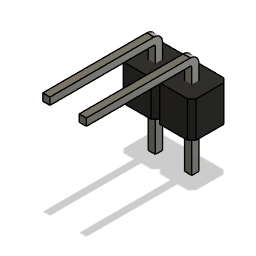
2.54mm 90 angle 2 pin header (Autodesk Fusion 360 design; units mm, degrees)
Autodesk Fusion 360 part; units mm, degrees
sketch "Sketch1" plane through (0, 0, 0) normal (0, 1, 0) x (1, 0, 0) in component "body"
  line L0 (0, 0) -> (-1.27, 0) construction
  line L1 (0, 0) -> (1.27, 0) construction
  line L2 (-0.0001, -1.27) -> (2.5401, -1.27)
  line L3 (2.5401, -1.27) -> (2.5401, 1.27)
  line L4 (2.5401, 1.27) -> (-0.0001, 1.27)
  line L5 (-0.0001, 1.27) -> (-0.0001, -1.27)
  line L6 (-0.0001, -1.27) -> (2.5401, 1.27) construction
  line L7 (2.5401, -1.27) -> (-0.0001, 1.27) construction
  line L8 (-0.0001, -1.27) -> (-2.5399, -1.27)
  line L9 (-2.5399, -1.27) -> (-2.5399, 1.27)
  line L10 (-2.5399, 1.27) -> (-0.0001, 1.27)
  line L11 (-0.0001, 1.27) -> (-0.0001, -1.27)
  line L12 (-0.0001, -1.27) -> (-2.5399, 1.27) construction
  line L13 (-2.5399, -1.27) -> (-0.0001, 1.27) construction
  point P0 (1.27, 0)
  point P1 (-1.27, 0)
  dimension "d1" = 1.27
  dimension "d2" = 1.27
  dimension "d3" = 2.54
  constraint coincident L0.start L1.start
  constraint horizontal L0
  constraint parallel L0 L1
  constraint horizontal L2
  constraint perpendicular L2 L3
  constraint parallel L2 L4
  constraint parallel L3 L5
  constraint coincident L6 P0
  constraint coincident L7 P0
  constraint coincident P0 L1.end
  constraint horizontal L8
  constraint perpendicular L8 L9
  constraint parallel L8 L10
  constraint parallel L9 L11
  constraint coincident L12 P1
  constraint coincident L13 P1
  constraint coincident P1 L0.end
  measures "d1" distance of L0.start L0.end
  measures "d2" distance of L0.start P0
  measures "d3" distance of L2.end L3.end
extrude "Extrude1" add sketch "Sketch1" along normal blind 2.5 contours L5 L8 L9 L10 L11 makes body 1 in component "body"
chamfer "Chamfer1" distance 0.3 angle 45 4 edges at (-0.0001, 1.25, 1.27) (-2.5399, 1.25, 1.27) (-0.0001, 1.25, -1.27) (-2.5399, 1.25, -1.27) on bodies 1 in component "body"
extrude "Extrude2" add sketch "Sketch1" along normal blind 2.5 contours L2 L3 L4 L5 L11 bodies 1 in component "body"
chamfer "Chamfer2" distance 0.3 angle 45 4 edges at (-0.0001, 1.25, 1.27) (2.5401, 1.25, 1.27) (2.5401, 1.25, -1.27) (-0.0001, 1.25, -1.27) on bodies 1 in component "body"
sketch "Sketch1 (2)" plane through (0, 2.5, 0) normal (0, 1, 0) x (-1, 0, 0) in component "pins"
  line L0 (-0.2999, -1.27) -> (0.0001, -0.97)
  line L1 (0.0001, -0.97) -> (0.3001, -1.27)
  line L2 (0.3001, -1.27) -> (2.2399, -1.27)
  line L3 (2.2399, -1.27) -> (2.5399, -0.97)
  line L4 (2.5399, -0.97) -> (2.5399, 0.97)
  line L5 (2.5399, 0.97) -> (2.2399, 1.27)
  line L6 (2.2399, 1.27) -> (0.3001, 1.27)
  line L7 (0.3001, 1.27) -> (0.0001, 0.97)
  line L8 (0.0001, 0.97) -> (-0.2999, 1.27)
  line L9 (-0.2999, 1.27) -> (-2.2401, 1.27)
  line L10 (-2.2401, 1.27) -> (-2.5401, 0.97)
  line L11 (-2.5401, 0.97) -> (-2.5401, -0.97)
  line L12 (-2.5401, -0.97) -> (-2.2401, -1.27)
  line L13 (-2.2401, -1.27) -> (-0.2999, -1.27)
  line L14 (-2.3901, -1.12) -> (-0.1499, 1.12) construction
  line L15 (0.1501, 1.12) -> (2.3899, -1.12) construction
  line L16 (-1.52, 0.25) -> (-1.02, 0.25)
  line L17 (-1.02, 0.25) -> (-1.02, -0.25)
  line L18 (-1.02, -0.25) -> (-1.52, -0.25)
  line L19 (-1.52, -0.25) -> (-1.52, 0.25)
  line L20 (-1.52, 0.25) -> (-1.02, -0.25) construction
  line L21 (-1.02, 0.25) -> (-1.52, -0.25) construction
  line L22 (1.02, 0.25) -> (1.52, 0.25)
  line L23 (1.52, 0.25) -> (1.52, -0.25)
  line L24 (1.52, -0.25) -> (1.02, -0.25)
  line L25 (1.02, -0.25) -> (1.02, 0.25)
  line L26 (1.02, 0.25) -> (1.52, -0.25) construction
  line L27 (1.52, 0.25) -> (1.02, -0.25) construction
  point P0 (-1.27, 0)
  point P1 (1.27, 0)
  dimension "d10" = 0.5
  dimension "d11" = 0.5
  constraint midpoint L12 L14.start
  constraint midpoint L8 L14.end
  constraint midpoint L7 L15.start
  constraint midpoint L3 L15.end
  constraint horizontal L16
  constraint perpendicular L16 L17
  constraint parallel L16 L18
  constraint parallel L17 L19
  constraint coincident L20 P0
  constraint coincident L21 P0
  constraint midpoint L14 P0
  constraint horizontal L22
  constraint perpendicular L22 L23
  constraint parallel L22 L24
  constraint parallel L23 L25
  constraint coincident L15 L22.start
  constraint coincident L26 P1
  constraint coincident L27 P1
  constraint midpoint L15 P1
  measures "d10" distance of L17.end L18.end
  measures "d11" distance of L16.end L17.end
extrude "Extrude1'" add sketch "Sketch1 (2)" against normal blind 5.5 separate body contours L16 L17 L18 L19 | L22 L23 L24 L25 makes body 2 at (1.02, 0.6667, 0.0833) makes body 3 at (-1.52, 0.6667, 0.0833) in component "pins"
sketch "Sketch2" plane through (2.5401, 0, 0) normal (1, 0, 0) x (0, 0, -1) in component "pins"
  line L0 (0.97, 0) -> (0.97, 2.5)
  line L1 (0.97, 2.5) -> (-0.97, 2.5)
  line L2 (-0.97, 2.5) -> (-0.97, 0)
  line L3 (-0.97, 0) -> (0.97, 0)
  line L4 (0, 2.5) -> (0, 3.55)
  line L5 (-0.35, 3.9) -> (-7.36, 3.9)
  line L6 (-7.36, 3.9) -> (-7.61, 3.9)
  arc A0 (0, 3.55) -> (-0.35, 3.9) centre (-0.35, 3.55) ccw
  point P0 (0, 2.5)
  point P1 (0, 3.9)
  dimension "d16" = 7.36
  dimension "d17" = 0.25
  dimension "d18" = 0.35
  constraint coincident P0 L4.start
  constraint perpendicular L1 L4
  constraint perpendicular L4 L5
  constraint parallel L5 L6
  constraint coincident L4 P1
  constraint coincident P1 L5
  constraint tangent L4 A0
  constraint tangent L5 A0
  measures "d16" distance of P1 L5.end
  measures "d17" distance of L5.end L6.end
  measures "d18" radius of A0
sweep "Sweep1" add profiles "Sketch1 (2)" path "Sketch2" along L4 A0 L5 L6 section 1 contours L16 L17 L18 L19 | L22 L23 L24 L25 bodies 2 3 in component "pins"
component "body" placed x (1, 0, 0) y (0, 1, 0) z (0, 0, 1) at (0, 0, 0)
component "pins" placed x (1, 0, 0) y (0, 1, 0) z (0, 0, 1) at (0, 0, 0)
